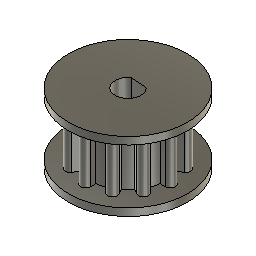
ZahnradMotor v5 (Autodesk Fusion 360 design; units mm, degrees)
Autodesk Fusion 360 part; units mm, degrees
sketch "Skizze1" plane through (0, 0, 0) normal (0, 0, 1) x (1, 0, 0)
  circle A0 centre (0, 0) radius 7.5541
  circle A1 centre (0, 8.5541) radius 1
  line L0 (-1, 8.5541) -> (1, 8.5541)
  line L1 (1, 8.5541) -> (1, 7.4877)
  line L2 (1, 7.4877) -> (-1, 7.4877)
  line L3 (-1, 7.4877) -> (-1, 8.5541)
  circle A2 centre (-4.2771, 7.4081) radius 1
  line L4 (-4.6099, 5.9845) -> (-5.1431, 6.9081)
  line L5 (-3.411, 7.9081) -> (-2.8778, 6.9845)
  circle A3 centre (-7.4081, 4.2771) radius 1
  line L6 (-6.9845, 2.8778) -> (-7.9081, 3.411)
  line L7 (-6.9081, 5.1431) -> (-5.9845, 4.6099)
  circle A4 centre (-8.5541, 0) radius 1
  line L8 (-7.4877, -1) -> (-8.5541, -1)
  line L9 (-8.5541, 1) -> (-7.4877, 1)
  circle A5 centre (-7.4081, -4.2771) radius 1
  line L10 (-5.9845, -4.6099) -> (-6.9081, -5.1431)
  line L11 (-7.9081, -3.411) -> (-6.9845, -2.8778)
  circle A6 centre (-4.2771, -7.4081) radius 1
  line L12 (-2.8778, -6.9845) -> (-3.411, -7.9081)
  line L13 (-5.1431, -6.9081) -> (-4.6099, -5.9845)
  circle A7 centre (0, -8.5541) radius 1
  line L14 (1, -7.4877) -> (1, -8.5541)
  line L15 (-1, -8.5541) -> (-1, -7.4877)
  circle A8 centre (4.2771, -7.4081) radius 1
  line L16 (4.6099, -5.9845) -> (5.1431, -6.9081)
  line L17 (3.411, -7.9081) -> (2.8778, -6.9845)
  circle A9 centre (7.4081, -4.2771) radius 1
  line L18 (6.9845, -2.8778) -> (7.9081, -3.411)
  line L19 (6.9081, -5.1431) -> (5.9845, -4.6099)
  circle A10 centre (8.5541, 0) radius 1
  line L20 (7.4877, 1) -> (8.5541, 1)
  line L21 (8.5541, -1) -> (7.4877, -1)
  circle A11 centre (7.4081, 4.2771) radius 1
  line L22 (5.9845, 4.6099) -> (6.9081, 5.1431)
  line L23 (7.9081, 3.411) -> (6.9845, 2.8778)
  circle A12 centre (4.2771, 7.4081) radius 1
  line L24 (2.8778, 6.9845) -> (3.411, 7.9081)
  line L25 (5.1431, 6.9081) -> (4.6099, 5.9845)
  circle A13 centre (0, 0) radius 12
  circle A14 centre (0, 0) radius 2.6
  line L26 (-1.5057, 2.1196) -> (1.8075, 1.869)
  circle A15 centre (0, 0) radius 9.5541
  dimension "d2" = 2
  dimension "d4" = 360
  dimension "d13" = 5.2
  dimension "d14" = 2
  dimension "d24" = 19.1083
  constraint coincident A0.centre A13.centre
  constraint tangent A0 A1
  constraint perpendicular L0 L1
  constraint parallel L0 L2
  constraint parallel L1 L3
  constraint coincident A1 L0.end
  constraint horizontal L0
  constraint coincident A1 L0.start
  constraint coincident A0 L2.end
  constraint coincident A0 L1.end
  constraint coincident A14 L26.start
  constraint coincident A14 L26.end
  constraint concentric A0 A15
  constraint tangent A1 A15
  constraint tangent A1 L3
  measures "d2" diameter of A1
  measures "d13" diameter of A14
  measures "d14" distance of A0.centre L26
  measures "d24" diameter of A15
extrude "Extrusion1" add sketch "Skizze1" along normal blind 11 contours A0 L2 | A0 A10 L21 | A0 A10 L20 | A10 | A0 A11 L23 | A0 A9 L18 | A0 A11 L22 | A11 | A0 A9 L19 | A9 | A12 | A8 | A0 A12 L25 | A0 A8 L16 | A0 A12 L24 | A1 L0 | A0 A8 L17 | A7 | A0 A1 L1 | A1 L0 | A0 A1 L3 | A2 | A0 A7 L15 | A0 A7 L14 | A6 | A0 L2 | A0 A2 L5 | A0 A2 L4 | A3 | A0 A6 L13 | A0 A6 L12 | A5 | A0 A3 L7 | A0 A3 L6 | A4 | A0 A5 L11 | A0 A5 L10 | A0 A4 L9 | A0 A4 L8 | A14 L26 | A14 L26
extrude "Extrusion5" add sketch "Skizze1" against normal blind 1.5 contours A0 L2 | A0 A10 L21 | A0 A10 L20 | A10 | A0 A10 L20 A11 L23 A15 | A0 A9 L18 A10 L21 A15 | A0 A11 L23 | A0 A9 L18 | A0 A11 L22 | A11 | A0 A9 L19 | A9 | A0 A11 L22 A12 L25 A15 | A0 A8 L16 A9 L19 A15 | A12 | A0 A1 L1 A12 L24 A15 | A0 A7 L14 A8 L17 A15 | A8 | A0 A12 L25 | A0 A8 L16 | A0 A12 L24 | A1 L0 | A0 A1 L3 A2 L5 A15 | A0 A8 L17 | A0 A6 L12 A7 L15 A15 | A7 | A0 A1 L1 | A1 L0 | A0 A1 L3 | A2 | A0 A2 L4 A3 L7 A15 | A0 A7 L15 | A0 A7 L14 | A0 A5 L10 A6 L13 A15 | A6 | A0 L2 | A0 A2 L5 | A0 A2 L4 | A3 | A0 A3 L6 A4 L9 A15 | A0 A6 L13 | A0 A6 L12 | A0 A4 L8 A5 L11 A15 | A5 | A0 A3 L7 | A0 A3 L6 | A4 | A0 A5 L11 | A0 A5 L10 | A0 A4 L9 | A0 A4 L8 | A13 | A14 L26 | A14 L26
extrude "Extrusion6" add sketch "Skizze1" 2 faces at (2.4283, 9.6405, 0) (2.4283, 9.6405, 0) along normal blind 1.5 contours A0 L2 | A0 A10 L21 | A0 A10 L20 | A10 | A0 A10 L20 A11 L23 A15 | A0 A9 L18 A10 L21 A15 | A0 A11 L23 | A0 A9 L18 | A0 A11 L22 | A11 | A0 A9 L19 | A9 | A0 A11 L22 A12 L25 A15 | A0 A8 L16 A9 L19 A15 | A12 | A0 A1 L1 A12 L24 A15 | A0 A7 L14 A8 L17 A15 | A8 | A0 A12 L25 | A0 A8 L16 | A0 A12 L24 | A1 L0 | A0 A1 L3 A2 L5 A15 | A0 A8 L17 | A0 A6 L12 A7 L15 A15 | A7 | A0 A1 L1 | A1 L0 | A0 A1 L3 | A2 | A0 A2 L4 A3 L7 A15 | A0 A7 L15 | A0 A7 L14 | A0 A5 L10 A6 L13 A15 | A6 | A0 L2 | A0 A2 L5 | A0 A2 L4 | A3 | A0 A3 L6 A4 L9 A15 | A0 A6 L13 | A0 A6 L12 | A0 A4 L8 A5 L11 A15 | A5 | A0 A3 L7 | A0 A3 L6 | A4 | A0 A5 L11 | A0 A5 L10 | A0 A4 L9 | A0 A4 L8 | A13 | A14 L26 | A14 L26 start surface through (0, 0, 11) normal (0, 0, 1)
extrude "Extrusion4" cut sketch "Skizze1" along normal up to surface (12.5 mm away) and the other way up to surface (1.5 mm away) contours A14 L26 picked at (-0.5022, 0.7068)
equation "d24 = ( 12 * 5 ) / 3.14 * 1 mm"
